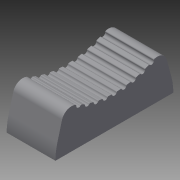
# Autodesk Inventor part: Finger_Handle
Saved by Autodesk Inventor 2015 (Build 190159000, 159)
## iProperties
Created: 2022-05-13
Part Number: Finger_Handle
Material: Generic
Document SubType Name: Modeling
Designer: Jan
Density: 1 g/cm^3
Appearance: Default
Author: Jan
Autodesk Inventor part; units mm, degrees
ref_plane "YZ Plane" through (0, 0, 0) normal (1, 0, 0) x (0, 1, 0)
ref_plane "XZ Plane" through (0, 0, 0) normal (0, 1, 0) x (-1, 0, 0)
ref_plane "XY Plane" through (0, 0, 0) normal (0, 0, 1) x (1, 0, 0)
sketch "Sketch1" plane through (0, 0, 0) normal (1, 0, 0) x (0, 1, 0)
  line L0 (12.5, 0) -> (-12.5, 0)
  line L1 (-12.5, 0) -> (-10.0674, 9.0786)
  line L2 (12.5, 0) -> (10.0674, 9.0786)
  line L3 (0, -7.32) -> (0, 29.22) construction
  arc A0 (-10.0674, 9.0786) -> (10.0674, 9.0786) centre (0, 24) ccw
  line L4 (-9.25, -2.1) -> (-9.25, 5.4) construction
  line L5 (-9.25, 5.4) -> (9.25, 5.4) construction
  line L6 (9.25, 5.4) -> (9.25, -2.1) construction
  line L7 (-9.25, -2.1) -> (9.25, -2.1) construction
  line L8 (-3.7239, 6) -> (3.9055, 6) construction
  arc A1 (12.0911, 0) -> (11.6962, 3) centre (0.5, 0) ccw
  arc A2 (-11.6962, 3) -> (-12.0911, 0) centre (-0.5, 0) ccw
  point P0 (0, 0)
  dimension "d3" = 75
  dimension "d4" = 18.5
  dimension "d6" = 25
  dimension "d7" = 7.5
  dimension "d8" = 6
  dimension "d9" = 5.4
  dimension "d10" = 18
  dimension "d14" = 3
  constraints: 16 end point, 7 point on line, 6 point on circle, 4 horizontal, 3 centre point, 3 tangent, 1 midpoint, 1 vertical, 3 other
  measures "d3" angle of L0 L1
  measures "d4" distance between parallel lines of L6 L4
  measures "d6" distance of L0.start L0.end
  measures "d7" distance between parallel lines of L7 L5
  measures "d8" distance between parallel lines of L0 L8
  measures "d9" distance between parallel lines of L0 L5
  measures "d10" radius of A0
  measures "d14" distance from line of L0 A2.start
extrude "Extrusion2" add sketch "Sketch1" along normal blind 10 contours L0 A2 L1 A0 L2 A1
fillet "Fillet1" radius 2 2 edges at (5, -10.0674, 9.0786) (5, 10.0674, 9.0786)
sketch "Sketch2" plane through (10, 0, 0) normal (1, 0, 0) x (0, 0, -1)
  arc A0 (-6.5625, 10.7416) -> (-7.8403, 7.9288) centre (-6.0448, 8.8097) ccw projected
  arc A1 (-7.8403, -7.9288) -> (-7.8403, 7.9288) centre (-24, 0) ccw projected
  arc A2 (-7.8403, -7.9288) -> (-6.5625, -10.7416) centre (-6.0448, -8.8097) ccw projected
  line L0 (-6.5625, -10.7416) -> (-3, -11.6962) projected
  arc A3 (-3, -11.6962) -> (0, -12.0911) centre (0, -0.5) ccw projected
  line L1 (0, -12.0911) -> (0, 12.0911) projected
  arc A4 (0, 12.0911) -> (-3, 11.6962) centre (0, 0.5) ccw projected
  line L2 (-3, 11.6962) -> (-6.5625, 10.7416) projected
  arc A5 (-7.8403, -7.9288) -> (-7.8403, 7.9288) centre (-24, 0) ccw projected
  circle A6 centre (-6, 0) radius 0.5
  circle A7 centre (-6.107, 1.9596) radius 0.5
  circle A8 centre (-6.4267, 3.8959) radius 0.5
  circle A9 centre (-6.9553, 5.7859) radius 0.5
  circle A10 centre (-7.6865, 7.6071) radius 0.5
  circle A11 centre (-6.0986, -1.8815) radius 0.5
  circle A12 centre (-6.3933, -3.7424) radius 0.5
  circle A13 centre (-6.881, -5.5623) radius 0.5
  circle A14 centre (-7.5562, -7.3213) radius 0.5
  point P0 (0, 0)
  dimension "d20" = 25
  dimension "d22" = 1
  dimension "d25" = 24
  constraints: 9 centre point, 2 point on circle, 18 other
  measures "d22" diameter of A6
extrude "Extrusion3" cut sketch "Sketch2" against normal up to next contours A10 A1 A0 | A0 A1 A10 | A9 A1 | A1 A9 | A8 A1 | A1 A8 | A7 A1 | A1 A7 | A14 A1 | A1 A14 | A6 A1 | A1 A6 | A13 A1 | A1 A13 | A11 A1 | A1 A11 | A12 A1 | A1 A12
fillet "Fillet2" radius 0.2 18 edges at (5, -7.7752, 7.7659) (5, -6.8617, 7.3592) (5, -6.0356, 7.0421) (5, -5.0847, 6.7331) (5, -4.23, 6.5041) (5, -3.2519, 6.2962) (5, -2.378, 6.1578) (5, -1.3836, 6.0533) (5, -0.5, 6.0069) (5, 0.5, 6.0069) (5, 1.4619, 6.0595) (5, 2.4558, 6.1683) (5, 3.4063, 6.3252) (5, 4.3825, 6.5417) (5, 6.2571, 7.1225) (5, 5.3103, 6.8011) (5, 7.1511, 7.4815) (5, 8.0598, 7.8989)
sketch "Sketch3" plane through (0, -12.0911, 0) normal (0, 0, -1) x (-1, 0, 0)
  line L0 (0, 0) -> (0, 24.1822) projected
  line L1 (0, 24.1822) -> (-10, 24.1822) projected
  line L2 (-10, 0) -> (-10, 24.1822) projected
  line L3 (0, 0) -> (-10, 0) projected
  line L4 (0, 0) -> (-10, 0) construction
  line L5 (-5, 0) -> (-5, 24.1822) construction
  line L6 (0, 24.1822) -> (-10, 24.1822) construction
  line L7 (0, 12.0911) -> (-10, 12.0911) construction
  line L8 (-10, 0) -> (-10, 24.1822) construction
  line L9 (-5.8, 2.5911) -> (-4.2, 2.5911)
  line L10 (-4.2, 2.5911) -> (-4.2, 21.5911)
  line L11 (-4.2, 21.5911) -> (-5.8, 21.5911)
  line L12 (-5.8, 21.5911) -> (-5.8, 2.5911)
  dimension "d30" = 19
  dimension "d31" = 1.6
  constraints: 12 end point, 3 midpoint, 2 parallel, 1 horizontal, 1 perpendicular, 2 other
  measures "d30" distance between parallel lines of L11 L9
  measures "d31" distance between parallel lines of L10 L12
extrude "Extrusion4" cut sketch "Sketch3" against normal blind 5 contours L12 L11 L10 L9
body "Solid2"
